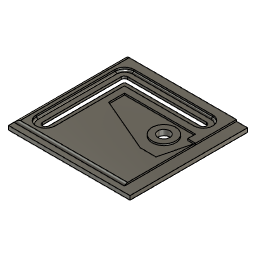
Body-Wall-E-Left_ (Autodesk Fusion 360 design; units mm, degrees)
Autodesk Fusion 360 part; units mm, degrees
sketch "Sketch1" plane through (0, 0, 0) normal (0, 0, 1) x (1, 0, 0)
  line L0 (0, 0) -> (-140, 0)
  line L1 (-140, 0) -> (-140, 140)
  line L2 (-140, 140) -> (0, 140)
  line L3 (0, 140) -> (0, 0)
  line L4 (-120, 110) -> (-20, 110)
  arc A0 (-20, 110) -> (-20, 130) centre (-20, 120) ccw
  line L5 (-20, 130) -> (-120, 130)
  arc A1 (-120, 130) -> (-120, 110) centre (-120, 120) ccw
  line L6 (-120, 120) -> (-20, 120) construction
  line L7 (-130, 120) -> (-130, 20)
  arc A2 (-130, 20) -> (-110, 20) centre (-120, 20) ccw
  line L8 (-110, 20) -> (-110, 120)
  arc A3 (-110, 120) -> (-130, 120) centre (-120, 120) ccw
  line L9 (-120, 120) -> (-120, 20) construction
  dimension "d1" = 140
  dimension "d2" = 140
  constraint horizontal L0
  constraint vertical L1
  constraint horizontal L2
  constraint vertical L3
  constraint coincident L0.start L3.end
  constraint tangent L4 A0
  constraint tangent A0 L5
  constraint parallel L4 L5
  constraint tangent L5 A1
  constraint tangent L4 A1
  constraint horizontal L6
  constraint tangent L7 A2
  constraint tangent A2 L8
  constraint parallel L7 L8
  constraint tangent L8 A3
  constraint tangent L7 A3
  constraint perpendicular L4 L9
  constraint coincident A1.centre L6.start
  measures "d1" distance of L0.start L0.end
  measures "d2" distance of L0.start L2.end
extrude "Extrude1" add sketch "Sketch1" along normal blind 3 contours L4 A1 L8 A3 | L4 A1 L7 A2 L8 | L4 A0 L5 L8 A3 makes body 1
extrude "Extrude2" add sketch "Sketch1" along normal blind 5 bodies 1
sketch "Sketch2" plane through (0, 0, 5) normal (0, 0, 1) x (-1, 0, 0)
  line L0 (120, -130) -> (20, -130)
  arc A0 (20, -110) -> (20, -130) centre (20, -120) ccw
  line L1 (20, -110) -> (110, -110)
  line L2 (110, -110) -> (110, -20)
  arc A1 (130, -20) -> (110, -20) centre (120, -20) ccw
  line L3 (130, -20) -> (130, -120)
  arc A2 (120, -130) -> (130, -120) centre (120, -120) ccw
  line L4 (0, -140) -> (140, -140)
  line L5 (140, -140) -> (140, 0)
  line L6 (140, 0) -> (0, 0)
  line L7 (0, 0) -> (0, -140)
  circle A3 centre (30, -80) radius 15
  dimension "d7" = 30
  measures "d7" diameter of A3
extrude "Extrude3" add sketch "Sketch2" along normal blind 2 contours A3 bodies 1
sketch "Sketch3" plane through (0, 0, 3) normal (0, 0, 1) x (-1, 0, 0)
  line L0 (20, -130) -> (120, -130)
  arc A0 (120, -130) -> (130, -120) centre (120, -120) ccw
  line L1 (130, -120) -> (130, -20)
  arc A1 (130, -20) -> (110, -20) centre (120, -20) ccw
  line L2 (110, -20) -> (110, -110)
  line L3 (110, -110) -> (20, -110)
  arc A2 (20, -110) -> (20, -130) centre (20, -120) ccw
  line L4 (120, -116) -> (20, -116)
  arc A3 (20, -116) -> (20, -124) centre (20, -120) ccw
  line L5 (20, -124) -> (120, -124)
  arc A4 (120, -124) -> (120, -116) centre (120, -120) ccw
  line L6 (120, -120) -> (20, -120) construction
  line L7 (124, -120) -> (124, -20)
  arc A5 (124, -20) -> (116, -20) centre (120, -20) ccw
  line L8 (116, -20) -> (116, -120)
  arc A6 (116, -120) -> (124, -120) centre (120, -120) ccw
  line L9 (120, -120) -> (120, -20) construction
  dimension "d10" = 8
  dimension "d11" = 8
  constraint tangent L4 A3
  constraint tangent A3 L5
  constraint parallel L4 L5
  constraint tangent L5 A4
  constraint tangent L4 A4
  constraint coincident A2.centre A3.centre
  constraint horizontal L6
  constraint coincident A0.centre A4.centre
  constraint tangent L7 A5
  constraint tangent A5 L8
  constraint parallel L7 L8
  constraint tangent L8 A6
  constraint tangent L7 A6
  constraint coincident A1.centre A5.centre
  constraint perpendicular L4 L9
  measures "d10" diameter of A3
  measures "d11" diameter of A5
extrude "Extrude4" cut sketch "Sketch3" against normal blind 5 contours L4 A4 L8 A6 | L4 A4 L7 A5 L8 | L4 A3 L5 L8 A6 bodies 1
fillet "Fillet1" radius 2 7 edges at (-110, 65, 5) (-120, 10, 5) (-130, 70, 5) (-127.0711, 127.0711, 5) (-70, 130, 5) (-10, 120, 5) (-65, 110, 5) on bodies 1
fillet "Fillet2" radius 2 1 edges at (-116, 116, 1.5) on bodies 1
sketch "Sketch4" plane through (0, 0, 5) normal (0, 0, 1) x (-1, 0, 0)
  line L0 (0, -140) -> (140, -140)
  line L1 (140, -140) -> (140, 0)
  line L2 (140, 0) -> (0, 0)
  line L3 (0, 0) -> (0, -140)
  circle A0 centre (30, -80) radius 15
  line L4 (108, -108) -> (108, -20)
  arc A1 (132, -20) -> (108, -20) centre (120, -20) ccw
  line L5 (132, -20) -> (132, -120)
  arc A2 (120, -132) -> (132, -120) centre (120, -120) ccw
  line L6 (120, -132) -> (20, -132)
  arc A3 (20, -108) -> (20, -132) centre (20, -120) ccw
  line L7 (20, -108) -> (108, -108)
  line L8 (100, -100) -> (10, -100)
  line L9 (10, -90) -> (10, -100)
  line L10 (10, -90) -> (0, -90)
  line L11 (0, -90) -> (10, -50)
  line L12 (10, -50) -> (30, -50)
  line L13 (30, -50) -> (100, -80)
  line L14 (100, -80) -> (100, -100)
  constraint horizontal L8
  constraint perpendicular L8 L9
  constraint coincident L3 L10.end
  constraint perpendicular L3 L10
  constraint perpendicular L3 L12
  constraint perpendicular L8 L14
extrude "Extrude5" add sketch "Sketch4" along normal blind 2 separate body contours L0 L1 L2 L3 makes body 2
fillet "Fillet3" radius 5 2 edges at (-140, 70, 7) (-70, 0, 7) on bodies 2
extrude "Extrude6" add 1 faces at (0, 93.3333, 3.3333) along direction (1, 0, 0) blind 7 on bodies 1 bodies 1 2
extrude "Extrude7" add 1 faces at (-44.3333, 0, 1.6667) along direction (0, -1, 0) blind 7 on bodies 1 bodies 1
extrude "Extrude8" add 1 faces at (-92, 140, 4) along direction (0, 1, 0) blind 7 on bodies 1 bodies 1
extrude "Extrude9" add 1 faces at (7, 44.3333, 1.6667) along direction (1, 0, 0) blind 7 on bodies 1 bodies 1
sketch "Sketch5" plane through (0, 0, 7) normal (0, 0, 1) x (-1, 0, 0)
  circle A0 centre (30, -80) radius 15
  circle A1 centre (30, -80) radius 7.5
  dimension "d30" = 15
  constraint concentric A0 A1
  measures "d30" diameter of A1
extrude "Extrude10" cut sketch "Sketch5" against normal blind 5 contours A1 bodies 1
extrude "Extrude11" cut 1 faces at (-29.4437, 77.783, 2) along direction (0, 0, -1) blind 45 on bodies 1 bodies 1
extrude "Extrude12" cut 1 faces at (-92, 147, 4) along direction (0, -1, 0) blind 5.032 on bodies 1 bodies 1
